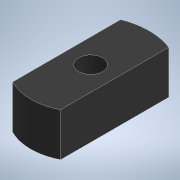
# Autodesk Inventor part: sHUFFLE
Saved by Autodesk Inventor 2021 (Build 250183000, 183)
## iProperties
Created: 2021-04-15
Part Number: sHUFFLE
Material: Generic
Document SubType Name: Modeling
Designer: calst
Density: 1 g/cm^3
Appearance: Rubber - Black
Author: calst
Autodesk Inventor part; units mm, degrees
ref_plane "YZ Plane" through (0, 0, 0) normal (1, 0, 0) x (0, 1, 0)
ref_plane "XZ Plane" through (0, 0, 0) normal (0, 1, 0) x (-1, 0, 0)
ref_plane "XY Plane" through (0, 0, 0) normal (0, 0, 1) x (1, 0, 0)
sketch "Sketch1" plane through (0, 0, 0) normal (0, 1, 0) x (-1, 0, 0)
  line L0 (0, 0) -> (5, 0)
  line L1 (5, 0) -> (5, 9.798)
  line L2 (5, 0) -> (5, -12.702)
  line L3 (-5, -12.702) -> (-5, 9.798)
  arc A0 (5, 9.798) -> (-5, 9.798) centre (0, 0) ccw
  arc A1 (-5, -12.702) -> (5, -12.702) centre (0, 0) ccw
  dimension "d1" = 5
  dimension "d7" = 22.5
  constraints: 8 end point, 4 point on circle, 2 centre point, 1 coincident, 1 horizontal, 1 parallel, 1 perpendicular, 1 point on line
  measures "d1" distance of L0.start L0.end
  measures "d7" distance of L2.end L1.end
extrude "Extrusion1" add sketch "Sketch1" along normal blind 9
sketch "Sketch2" plane through (0, 0, 0) normal (0, -1, 0) x (1, 0, 0)
  line L0 (-5, -12.702) -> (-5, 9.798) projected
  line L1 (-5, -12.702) -> (-5, -1.452)
  circle A0 centre (0, -1.452) radius 2.5
  point P0 (0, 0)
  dimension "d8" = 11.25
  dimension "d9" = 5
  constraints: 2 end point, 1 centre point, 1 midpoint
  measures "d8" distance of L0.start L1.end
  measures "d9" diameter of A0
extrude "Extrusion3" cut sketch "Sketch2" against normal blind 9
body "Solid1"
